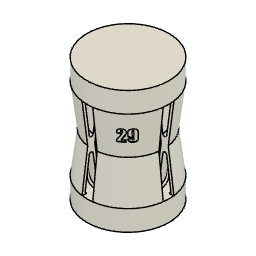
Cylinder design 3_Perez Leonardo v7 (Autodesk Fusion 360 design; units mm, degrees)
Autodesk Fusion 360 part; units mm, degrees
sketch "Sketch1" plane through (0, 0, 0) normal (0, 0, 1) x (1, 0, 0)
  line L0 (-12.7, 0) -> (12.7, 0)
  line L1 (12.7, 0) -> (12.7, 38.1)
  line L2 (12.7, 38.1) -> (-12.7, 38.1)
  line L3 (-12.7, 38.1) -> (-12.7, 0)
  line L4 (-12.7, 6.35) -> (12.7, 6.35)
  line L5 (-12.7, 31.75) -> (12.7, 31.75)
  line L6 (0, 0) -> (0, 38.1)
  line L7 (2.54, 6.35) -> (-2.54, 6.35)
  line L8 (-2.54, 6.35) -> (-2.54, 31.75)
  line L9 (-2.54, 31.75) -> (2.54, 31.75)
  line L10 (2.54, 31.75) -> (2.54, 6.35)
  line L11 (-7.62, 6.35) -> (-7.62, 31.75) construction
  line L12 (7.62, 6.35) -> (7.62, 31.75) construction
  line L13 (12.7, 19.05) -> (-12.7, 19.05) construction
  line L14 (-12.7, 6.35) -> (-11.1402, 19.0534)
  line L15 (-12.7, 6.35) -> (0.0988, 6.35) construction
  line L16 (-7.62, 6.35) -> (-9.1794, 19.05)
  line L17 (-7.62, 6.35) -> (-20.4154, 6.35) construction
  line L18 (-8.3877, 6.35) -> (-20.4994, 6.35) construction
  line L19 (-11.9323, 6.35) -> (0.0739, 6.35) construction
  line L20 (-8.3877, 6.35) -> (-9.6352, 16.51)
  line L21 (-11.9323, 6.35) -> (-10.6848, 16.51)
  line L22 (-11.9323, 31.75) -> (-10.6848, 21.59)
  line L23 (-8.3877, 31.75) -> (-9.6352, 21.59)
  line L24 (-7.62, 31.75) -> (-9.1794, 19.05)
  line L25 (-12.7, 31.75) -> (-11.1402, 19.0466)
  line L26 (-3.3077, 31.75) -> (-4.5552, 21.59)
  line L27 (-2.54, 31.75) -> (-4.0998, 19.0466)
  line L28 (-6.8523, 31.75) -> (-5.6048, 21.59)
  line L29 (-7.62, 31.75) -> (-6.0606, 19.05)
  line L30 (-2.54, 6.35) -> (-4.0998, 19.0534)
  line L31 (-7.62, 6.35) -> (-6.0606, 19.05)
  line L32 (-6.8523, 6.35) -> (-5.6048, 16.51)
  line L33 (-3.3077, 6.35) -> (-4.5552, 16.51)
  line L34 (12.7, 31.75) -> (11.1402, 19.0466)
  line L35 (11.9323, 31.75) -> (10.6848, 21.59)
  line L36 (8.3877, 31.75) -> (9.6352, 21.59)
  line L37 (7.62, 31.75) -> (9.1794, 19.05)
  line L38 (7.62, 31.75) -> (6.0606, 19.05)
  line L39 (6.8523, 31.75) -> (5.6048, 21.59)
  line L40 (3.3077, 31.75) -> (4.5552, 21.59)
  line L41 (2.54, 31.75) -> (4.0998, 19.0466)
  line L42 (2.54, 6.35) -> (4.0998, 19.0534)
  line L43 (3.3077, 6.35) -> (4.5552, 16.51)
  line L44 (6.8523, 6.35) -> (5.6048, 16.51)
  line L45 (7.62, 6.35) -> (6.0606, 19.05)
  line L46 (7.62, 6.35) -> (9.1794, 19.05)
  line L47 (8.3877, 6.35) -> (9.6352, 16.51)
  line L48 (11.9323, 6.35) -> (10.6848, 16.51)
  line L49 (12.7, 6.35) -> (11.1402, 19.0534)
  arc A0 (-9.6391, 16.51) -> (-10.6809, 16.51) centre (-10.16, 16.51) ccw
  line L50 (-10.6848, 16.51) -> (-10.6809, 16.51)
  line L51 (-9.6391, 16.51) -> (-9.6352, 16.51)
  arc A1 (-11.8606, 6.9342) -> (-11.3437, 6.35) centre (-11.3437, 6.8707) ccw
  arc A2 (-4.5591, 16.51) -> (-5.6009, 16.51) centre (-5.08, 16.51) ccw
  line L52 (-4.5552, 16.51) -> (-4.5591, 16.51)
  line L53 (-5.6009, 16.51) -> (-5.6048, 16.51)
  arc A3 (5.6009, 16.51) -> (4.5591, 16.51) centre (5.08, 16.51) ccw
  line L54 (4.5552, 16.51) -> (4.5591, 16.51)
  line L55 (5.6009, 16.51) -> (5.6048, 16.51)
  arc A4 (10.6809, 16.51) -> (9.6391, 16.51) centre (10.16, 16.51) ccw
  line L56 (10.6848, 16.51) -> (10.6809, 16.51)
  line L57 (9.6391, 16.51) -> (9.6352, 16.51)
  arc A5 (-8.9763, 6.35) -> (-8.4594, 6.9342) centre (-8.9763, 6.8707) ccw
  arc A6 (-6.7806, 6.9342) -> (-6.2637, 6.35) centre (-6.2637, 6.8707) ccw
  arc A7 (-3.8963, 6.35) -> (-3.3794, 6.9342) centre (-3.8963, 6.8707) ccw
  arc A8 (3.3794, 6.9342) -> (3.8963, 6.35) centre (3.8963, 6.8707) ccw
  arc A9 (6.2637, 6.35) -> (6.7806, 6.9342) centre (6.2637, 6.8707) ccw
  arc A10 (8.4594, 6.9342) -> (8.9763, 6.35) centre (8.9763, 6.8707) ccw
  arc A11 (11.3437, 6.35) -> (11.8606, 6.9342) centre (11.3437, 6.8707) ccw
  arc A12 (-10.6809, 21.59) -> (-9.6391, 21.59) centre (-10.16, 21.59) ccw
  line L58 (-10.6848, 21.59) -> (-10.6809, 21.59)
  line L59 (-9.6391, 21.59) -> (-9.6352, 21.59)
  line L60 (-4.5552, 21.59) -> (-4.5591, 21.59)
  line L61 (-5.6009, 21.59) -> (-5.6048, 21.59)
  arc A13 (-5.6009, 21.59) -> (-4.5591, 21.59) centre (-5.08, 21.59) ccw
  line L62 (4.5552, 21.59) -> (4.5591, 21.59)
  line L63 (5.6009, 21.59) -> (5.6048, 21.59)
  arc A14 (4.5591, 21.59) -> (5.6009, 21.59) centre (5.08, 21.59) ccw
  line L64 (10.6848, 21.59) -> (10.6809, 21.59)
  line L65 (9.6391, 21.59) -> (9.6352, 21.59)
  arc A15 (9.6391, 21.59) -> (10.6809, 21.59) centre (10.16, 21.59) ccw
  arc A16 (11.8606, 31.1658) -> (11.3437, 31.75) centre (11.3437, 31.2293) ccw
  arc A17 (8.9763, 31.75) -> (8.4594, 31.1658) centre (8.9763, 31.2293) ccw
  arc A18 (6.7806, 31.1658) -> (6.2637, 31.75) centre (6.2637, 31.2293) ccw
  arc A19 (3.8963, 31.75) -> (3.3794, 31.1658) centre (3.8963, 31.2293) ccw
  arc A20 (-3.3794, 31.1658) -> (-3.8963, 31.75) centre (-3.8963, 31.2293) ccw
  arc A21 (-6.2637, 31.75) -> (-6.7806, 31.1658) centre (-6.2637, 31.2293) ccw
  arc A22 (-8.4594, 31.1658) -> (-8.9763, 31.75) centre (-8.9763, 31.2293) ccw
  arc A23 (-11.3437, 31.75) -> (-11.8606, 31.1658) centre (-11.3437, 31.2293) ccw
  circle A24 centre (-7.62, 26.5395) radius 0.635
  circle A25 centre (-7.62, 11.5605) radius 0.635
  circle A26 centre (7.62, 11.5605) radius 0.635
  circle A27 centre (7.62, 26.5395) radius 0.635
  dimension "d1" = 25.4
  dimension "d2" = 38.1
  dimension "d3" = 6.35
  dimension "d4" = 6.35
  dimension "d5" = 25.4
  dimension "d6" = 5.08
  dimension "d7" = 5.08
  dimension "d8" = 5.08
  dimension "d9" = 83
  dimension "d10" = 83
  dimension "d11" = 83
  dimension "d12" = 83
  dimension "d13" = 0.762
  dimension "d14" = 0.762
  dimension "d15" = 10.16
  dimension "d17" = 1.0417
  dimension "d18" = 1.0414
  dimension "d49" = 1.27
  constraint horizontal L0
  constraint vertical L1
  constraint horizontal L2
  constraint vertical L3
  constraint midpoint L6.start L0
  constraint coincident L3 L4.start
  constraint coincident L1 L4.end
  constraint perpendicular L1 L4
  constraint coincident L3 L5.start
  constraint coincident L1 L5.end
  constraint perpendicular L1 L5
  constraint coincident L6.start origin
  constraint midpoint L2 L6.end
  constraint horizontal L7
  constraint vertical L8
  constraint horizontal L9
  constraint vertical L10
  constraint midpoint L4 L7
  constraint coincident L4 L11.start
  constraint coincident L5 L11.end
  constraint perpendicular L5 L11
  constraint coincident L4 L12.start
  constraint coincident L5 L12.end
  constraint perpendicular L5 L12
  constraint midpoint L1 L13.start
  constraint midpoint L3 L13.end
  constraint horizontal L15
  constraint horizontal L17
  constraint coincident L13 L16.end
  constraint horizontal L18
  constraint coincident L4 L18.start
  constraint horizontal L19
  constraint coincident L18 L19.start
  constraint perpendicular L11 L50
  constraint symmetric L4.start L13 L5.start
  constraint symmetric L11.start L13 L11.end
  constraint symmetric L13 L14.end L25.end
  constraint symmetric L13 L16.end L24.end
  constraint symmetric L13 L18.start L23.start
  constraint symmetric L13 L19.start L22.start
  constraint symmetric L13 L21.end L22.end
  constraint symmetric L13 L20.end L23.end
  constraint symmetric L4.start L11 L7.end
  constraint symmetric L16.start L11 L17.start
  constraint symmetric L11 L14.end L30.end
  constraint symmetric L11 L16.end L29.end
  constraint symmetric L11 L18.start L32.start
  constraint symmetric L11 L19.start L33.start
  constraint symmetric L11 L21.end L33.end
  constraint symmetric L11 L20.end L32.end
  constraint symmetric L11 L22.start L26.start
  constraint symmetric L11 L22.end L26.end
  constraint symmetric L11 L23.end L28.end
  constraint symmetric L11 L23.start L28.start
  constraint symmetric L11 L24.start L29.start
  constraint symmetric L11 L5.start L8.end
  constraint symmetric L11 L25.end L27.end
  constraint symmetric L4.start L6 L4.end
  constraint symmetric L6 L11.start L12.start
  constraint symmetric L6 L14.end L49.end
  constraint symmetric L6 L16.end L37.end
  constraint symmetric L6 L18.start L47.start
  constraint symmetric L6 L19.start L48.start
  constraint symmetric L6 L21.end L48.end
  constraint symmetric L6 L20.end L47.end
  constraint symmetric L6 L22.start L35.start
  constraint symmetric L6 L22.end L35.end
  constraint symmetric L6 L23.end L36.end
  constraint symmetric L6 L23.start L36.start
  constraint symmetric L6 L11.end L12.end
  constraint symmetric L6 L5.start L5.end
  constraint symmetric L6 L25.end L34.end
  constraint symmetric L6 L26.start L40.start
  constraint symmetric L6 L26.end L40.end
  constraint symmetric L6 L8.end L9.end
  constraint symmetric L6 L27.end L41.end
  constraint symmetric L6 L28.start L39.start
  constraint symmetric L6 L28.end L39.end
  constraint symmetric L6 L29.end L38.end
  constraint symmetric L6 L7.end L7.start
  constraint symmetric L6 L30.end L42.end
  constraint symmetric L6 L32.start L44.start
  constraint symmetric L6 L32.end L44.end
  constraint symmetric L6 L33.start L43.start
  constraint symmetric L6 L33.end L43.end
  constraint tangent L20 A0
  constraint tangent L21 A0
  constraint tangent L21 A1
  constraint tangent L17 A1
  constraint tangent L20 A5
  constraint tangent L18 A5
  constraint equal A1 A5
  constraint symmetric L11 A0 A2
  constraint symmetric L11 A1 A7
  constraint symmetric L11 A5 A6
  constraint symmetric L13 A0 A12
  constraint symmetric L13 A1 A23
  constraint symmetric L13 A5 A22
  constraint symmetric L13 A2 A13
  constraint symmetric L13 A7 A20
  constraint symmetric L13 A6 A21
  constraint symmetric L6 A0 A4
  constraint symmetric L6 A1 A11
  constraint symmetric L6 A5 A10
  constraint symmetric L6 A2 A3
  constraint symmetric L6 A7 A8
  constraint symmetric L6 A6 A9
  constraint symmetric L6 A18 A21
  constraint symmetric L6 A17 A22
  constraint symmetric L6 A16 A23
  constraint symmetric L6 A12 A15
  constraint symmetric L6 A13 A14
  constraint symmetric L6 A19 A20
  constraint coincident A0.start L50
  constraint collinear L50 L51
  constraint coincident A0.centre L50
  constraint coincident L4 A1.end
  constraint coincident L21 A1.start
  constraint coincident A2.end L52
  constraint collinear L52 L53
  constraint coincident A3.start L54
  constraint collinear L54 L55
  constraint coincident A4.end L56
  constraint collinear L56 L57
  constraint coincident L20 A5.end
  constraint coincident L4 A5.start
  constraint coincident L4 A6.end
  constraint coincident L32 A6.start
  constraint coincident L33 A7.end
  constraint coincident L4 A7.start
  constraint coincident L4 A8.end
  constraint coincident L43 A8.start
  constraint coincident L44 A9.end
  constraint coincident L4 A9.start
  constraint coincident L4 A10.end
  constraint coincident L47 A10.start
  constraint coincident L48 A11.end
  constraint coincident L4 A11.start
  constraint coincident A12.end L58
  constraint collinear L58 L59
  constraint collinear L60 L61
  constraint collinear L62 L63
  constraint collinear L64 L65
  constraint coincident L5 A16.end
  constraint coincident L35 A16.start
  constraint coincident L36 A17.end
  constraint coincident L5 A17.start
  constraint coincident L5 A18.end
  constraint coincident L39 A18.start
  constraint coincident L40 A19.end
  constraint coincident L5 A19.start
  constraint coincident L5 A20.end
  constraint coincident L26 A20.start
  constraint coincident L28 A21.end
  constraint coincident L5 A21.start
  constraint coincident L5 A22.end
  constraint coincident L23 A22.start
  constraint coincident L22 A23.end
  constraint coincident L5 A23.start
  constraint tangent L29 A24
  constraint tangent L24 A24
  constraint tangent L31 A25
  constraint tangent L16 A25
  constraint equal A24 A25
  constraint tangent L46 A26
  constraint tangent L45 A26
  constraint equal A25 A26
  constraint tangent L37 A27
  constraint tangent L38 A27
  constraint equal A26 A27
  measures "d1" distance of L0.start L0.end
  measures "d2" distance of L0.end L1.end
  measures "d3" distance of L2 L5
  measures "d4" distance of L0 L4
  measures "d5" distance of L7.start L9.end
  measures "d6" distance of L7.start L7.end
  measures "d7" distance of L8 L11
  measures "d8" distance of L10 L12
  measures "d9" angle of L14 L15
  measures "d10" angle of L16 L17
  measures "d11" angle of L18 L20
  measures "d12" angle of L19 L21
  measures "d13" distance of L14 L21
  measures "d14" distance of L16 L20
  measures "d15" distance of L4 L50
  measures "d17" diameter of A0
  measures "d18" diameter of A1
  measures "d49" diameter of A24
sketch "Sketch2" plane through (0, 0, 0) normal (1, 0, 0) x (0, 0, -1)
  line L0 (-7.62, 6.35) -> (-20.4154, 6.35) construction
  line L1 (-8.3877, 6.35) -> (-9.6352, 16.51)
  line L2 (-9.6391, 16.51) -> (-9.6352, 16.51)
  line L3 (-11.9323, 6.35) -> (-10.6848, 16.51)
  arc A0 (-4.5591, 16.51) -> (-5.6009, 16.51) centre (-5.08, 16.51) ccw
  arc A1 (-6.7806, 6.9342) -> (-6.2637, 6.35) centre (-6.2637, 6.8707) ccw
  arc A2 (-11.8606, 6.9342) -> (-11.3437, 6.35) centre (-11.3437, 6.8707) ccw
  arc A3 (-8.9763, 6.35) -> (-8.4594, 6.9342) centre (-8.9763, 6.8707) ccw
  line L4 (-4.5552, 16.51) -> (-4.5591, 16.51)
  arc A4 (6.2637, 6.35) -> (6.7806, 6.9342) centre (6.2637, 6.8707) ccw
  arc A5 (10.6809, 16.51) -> (9.6391, 16.51) centre (10.16, 16.51) ccw
  arc A6 (11.8606, 31.1658) -> (11.3437, 31.75) centre (11.3437, 31.2293) ccw
  line L5 (3.3077, 6.35) -> (4.5552, 16.51)
  line L6 (6.8523, 6.35) -> (5.6048, 16.51)
  line L7 (-2.54, 6.35) -> (-4.0998, 19.0534)
  line L8 (5.6009, 21.59) -> (5.6048, 21.59)
  line L9 (-7.62, 6.35) -> (-6.0606, 19.05)
  line L10 (4.5552, 16.51) -> (4.5591, 16.51)
  arc A7 (6.7806, 31.1658) -> (6.2637, 31.75) centre (6.2637, 31.2293) ccw
  arc A8 (5.6009, 16.51) -> (4.5591, 16.51) centre (5.08, 16.51) ccw
  line L11 (11.9323, 31.75) -> (10.6848, 21.59)
  line L12 (9.6391, 16.51) -> (9.6352, 16.51)
  line L13 (7.62, 31.75) -> (9.1794, 19.05)
  line L14 (2.54, 31.75) -> (2.54, 6.35)
  line L15 (5.6009, 16.51) -> (5.6048, 16.51)
  line L16 (3.3077, 31.75) -> (4.5552, 21.59)
  arc A9 (8.4594, 6.9342) -> (8.9763, 6.35) centre (8.9763, 6.8707) ccw
  line L17 (-12.7, 6.35) -> (-11.1402, 19.0534)
  line L18 (12.7, 6.35) -> (11.1402, 19.0534)
  line L19 (10.6848, 16.51) -> (10.6809, 16.51)
  line L20 (2.54, 6.35) -> (4.0998, 19.0534)
  arc A10 (4.5591, 21.59) -> (5.6009, 21.59) centre (5.08, 21.59) ccw
  arc A11 (3.8963, 31.75) -> (3.3794, 31.1658) centre (3.8963, 31.2293) ccw
  line L21 (6.8523, 31.75) -> (5.6048, 21.59)
  line L22 (7.62, 6.35) -> (9.1794, 19.05)
  line L23 (8.3877, 31.75) -> (9.6352, 21.59)
  line L24 (10.6848, 21.59) -> (10.6809, 21.59)
  line L25 (-2.54, 6.35) -> (-2.54, 31.75)
  line L26 (11.9323, 6.35) -> (10.6848, 16.51)
  line L27 (8.3877, 6.35) -> (9.6352, 16.51)
  arc A12 (9.6391, 21.59) -> (10.6809, 21.59) centre (10.16, 21.59) ccw
  arc A13 (8.9763, 31.75) -> (8.4594, 31.1658) centre (8.9763, 31.2293) ccw
  line L28 (7.62, 31.75) -> (6.0606, 19.05)
  line L29 (2.54, 31.75) -> (4.0998, 19.0466)
  line L30 (7.62, 6.35) -> (6.0606, 19.05)
  line L31 (9.6391, 21.59) -> (9.6352, 21.59)
  line L32 (4.5552, 21.59) -> (4.5591, 21.59)
  line L33 (7.62, 6.35) -> (7.62, 31.75) construction
  line L34 (12.7, 0) -> (12.7, 38.1)
  arc A14 (3.3794, 6.9342) -> (3.8963, 6.35) centre (3.8963, 6.8707) ccw
  arc A15 (11.3437, 6.35) -> (11.8606, 6.9342) centre (11.3437, 6.8707) ccw
  line L35 (0, 0) -> (0, 38.1)
  line L36 (-12.7, 38.1) -> (-12.7, 0)
  line L37 (-6.8523, 6.35) -> (-5.6048, 16.51)
  line L38 (-6.8523, 31.75) -> (-5.6048, 21.59)
  arc A16 (-8.4594, 31.1658) -> (-8.9763, 31.75) centre (-8.9763, 31.2293) ccw
  line L39 (-4.5552, 21.59) -> (-4.5591, 21.59)
  arc A17 (-5.6009, 21.59) -> (-4.5591, 21.59) centre (-5.08, 21.59) ccw
  line L40 (-3.3077, 31.75) -> (-4.5552, 21.59)
  line L41 (-9.6391, 21.59) -> (-9.6352, 21.59)
  line L42 (-8.3877, 6.35) -> (-20.4994, 6.35) construction
  line L43 (-7.62, 31.75) -> (-6.0606, 19.05)
  arc A18 (-11.3437, 31.75) -> (-11.8606, 31.1658) centre (-11.3437, 31.2293) ccw
  line L44 (-2.54, 31.75) -> (-4.0998, 19.0466)
  arc A19 (-3.8963, 6.35) -> (-3.3794, 6.9342) centre (-3.8963, 6.8707) ccw
  line L45 (-7.62, 31.75) -> (-9.1794, 19.05)
  line L46 (-12.7, 31.75) -> (-11.1402, 19.0466)
  line L47 (-11.9323, 31.75) -> (-10.6848, 21.59)
  arc A20 (-10.6809, 21.59) -> (-9.6391, 21.59) centre (-10.16, 21.59) ccw
  line L48 (-3.3077, 6.35) -> (-4.5552, 16.51)
  arc A21 (-9.6391, 16.51) -> (-10.6809, 16.51) centre (-10.16, 16.51) ccw
  line L49 (-8.3877, 31.75) -> (-9.6352, 21.59)
  arc A22 (-3.3794, 31.1658) -> (-3.8963, 31.75) centre (-3.8963, 31.2293) ccw
  line L50 (-10.6848, 21.59) -> (-10.6809, 21.59)
  line L51 (-5.6009, 16.51) -> (-5.6048, 16.51)
  line L52 (-10.6848, 16.51) -> (-10.6809, 16.51)
  line L53 (-5.6009, 21.59) -> (-5.6048, 21.59)
  arc A23 (-6.2637, 31.75) -> (-6.7806, 31.1658) centre (-6.2637, 31.2293) ccw
  line L54 (-7.62, 6.35) -> (-9.1794, 19.05)
  line L55 (-7.62, 6.35) -> (-7.62, 31.75) construction
  line L56 (-12.7, 6.35) -> (0.0988, 6.35) construction
  line L57 (2.54, 6.35) -> (-2.54, 6.35)
  line L58 (12.7, 31.75) -> (11.1402, 19.0466)
  line L59 (12.7, 38.1) -> (-12.7, 38.1)
  line L60 (-2.54, 31.75) -> (2.54, 31.75)
  line L61 (-12.7, 0) -> (12.7, 0)
  line L62 (-12.7, 31.75) -> (12.7, 31.75)
  line L63 (-11.9323, 6.35) -> (0.0739, 6.35) construction
  line L64 (12.7, 19.05) -> (-12.7, 19.05) construction
  line L65 (-12.7, 6.35) -> (12.7, 6.35)
  circle A24 centre (-7.62, 26.5395) radius 0.635
  circle A25 centre (-7.62, 11.5605) radius 0.635
  circle A26 centre (7.62, 26.5395) radius 0.635
  circle A27 centre (7.62, 11.5605) radius 0.635
  dimension "d20" = 25.4
  dimension "d21" = 38.1
  dimension "d22" = 6.35
  dimension "d23" = 6.35
  dimension "d24" = 25.4
  dimension "d25" = 5.08
  dimension "d26" = 5.08
  dimension "d27" = 5.08
  dimension "d28" = 83
  dimension "d29" = 83
  dimension "d30" = 83
  dimension "d31" = 83
  dimension "d32" = 0.762
  dimension "d33" = 0.762
  dimension "d34" = 10.16
  dimension "d35" = 1.0417
  dimension "d36" = 1.0414
  dimension "d37" = 12.7
  dimension "d50" = 1.27
  constraint horizontal L61
  constraint vertical L34
  constraint horizontal L59
  constraint vertical L36
  constraint midpoint L35.start L61
  constraint coincident L17.start L36
  constraint coincident L18.start L34
  constraint perpendicular L34 L65
  constraint coincident L46.start L36
  constraint coincident L58.start L34
  constraint perpendicular L34 L62
  constraint coincident L35.start origin
  constraint midpoint L35.end L59
  constraint horizontal L57
  constraint vertical L25
  constraint horizontal L60
  constraint vertical L14
  constraint midpoint L57 L65
  constraint coincident L0.start L65
  constraint coincident L43.start L62
  constraint perpendicular L55 L62
  constraint coincident L22.start L65
  constraint coincident L13.start L62
  constraint perpendicular L33 L62
  constraint midpoint L64.start L34
  constraint midpoint L64.end L36
  constraint horizontal L56
  constraint horizontal L0
  constraint coincident L45.end L64
  constraint horizontal L42
  constraint coincident L1.start L65
  constraint horizontal L63
  constraint coincident L3.start L42
  constraint perpendicular L52 L55
  constraint symmetric L17.start L46.start L64
  constraint symmetric L0.start L43.start L64
  constraint symmetric L17.end L46.end L64
  constraint symmetric L45.end L54.end L64
  constraint symmetric L1.start L49.start L64
  constraint symmetric L3.start L47.start L64
  constraint symmetric L3.end L47.end L64
  constraint symmetric L1.end L41.end L64
  constraint symmetric L17.start L7.start L55
  constraint symmetric L0.start L9.start L55
  constraint symmetric L17.end L7.end L55
  constraint symmetric L45.end L9.end L55
  constraint symmetric L1.start L37.start L55
  constraint symmetric L3.start L48.start L55
  constraint symmetric L3.end L4.start L55
  constraint symmetric L1.end L37.end L55
  constraint symmetric L47.start L40.start L55
  constraint symmetric L47.end L39.start L55
  constraint symmetric L41.end L38.end L55
  constraint symmetric L49.start L38.start L55
  constraint symmetric L43.start L45.start L55
  constraint symmetric L25.end L46.start L55
  constraint symmetric L46.end L44.end L55
  constraint symmetric L17.start L18.start L35
  constraint symmetric L0.start L22.start L35
  constraint symmetric L17.end L18.end L35
  constraint symmetric L45.end L13.end L35
  constraint symmetric L1.start L27.start L35
  constraint symmetric L3.start L26.start L35
  constraint symmetric L3.end L19.start L35
  constraint symmetric L1.end L12.end L35
  constraint symmetric L47.start L11.start L35
  constraint symmetric L47.end L11.end L35
  constraint symmetric L41.end L23.end L35
  constraint symmetric L49.start L23.start L35
  constraint symmetric L43.start L13.start L35
  constraint symmetric L46.start L58.start L35
  constraint symmetric L46.end L58.end L35
  constraint symmetric L40.start L16.start L35
  constraint symmetric L39.start L16.end L35
  constraint symmetric L25.end L14.start L35
  constraint symmetric L44.end L29.end L35
  constraint symmetric L38.start L21.start L35
  constraint symmetric L38.end L8.end L35
  constraint symmetric L9.end L28.end L35
  constraint symmetric L7.start L14.end L35
  constraint symmetric L7.end L20.end L35
  constraint symmetric L37.start L6.start L35
  constraint symmetric L37.end L6.end L35
  constraint symmetric L48.start L5.start L35
  constraint symmetric L4.start L5.end L35
  constraint tangent L1 A21
  constraint tangent L3 A21
  constraint tangent L3 A2
  constraint tangent L0 A2
  constraint tangent L1 A3
  constraint tangent A3 L42
  constraint equal A2 A3
  constraint symmetric A0 A21 L55
  constraint symmetric A2 A19 L55
  constraint symmetric A1 A3 L55
  constraint symmetric A20 A21 L64
  constraint symmetric A2 A18 L64
  constraint symmetric A3 A16 L64
  constraint symmetric A0 A17 L64
  constraint symmetric A19 A22 L64
  constraint symmetric A1 A23 L64
  constraint symmetric A5 L35 A21
  constraint symmetric A2 A15 L35
  constraint symmetric A3 A9 L35
  constraint symmetric A0 A8 L35
  constraint symmetric A14 L35 A19
  constraint symmetric A1 A4 L35
  constraint symmetric A7 L35 A23
  constraint symmetric A13 L35 A16
  constraint symmetric A6 L35 A18
  constraint symmetric A12 L35 A20
  constraint symmetric A10 L35 A17
  constraint symmetric A11 L35 A22
  constraint coincident L2.start L52
  constraint collinear L2 L52
  constraint coincident A21.centre L52
  constraint coincident A2.end L65
  constraint coincident A2.start L3
  constraint coincident A0.end L4
  constraint collinear L4 L51
  constraint coincident A8.start L10
  constraint collinear L10 L15
  constraint coincident A5.end L19
  constraint collinear L12 L19
  constraint coincident A3.end L1
  constraint coincident A3.start L65
  constraint coincident A1.end L65
  constraint coincident A1.start L37
  constraint coincident A19.end L48
  constraint coincident A19.start L65
  constraint coincident A14.end L65
  constraint coincident A14.start L5
  constraint coincident A4.end L6
  constraint coincident A4.start L65
  constraint coincident A9.end L65
  constraint coincident A9.start L27
  constraint coincident A15.end L26
  constraint coincident A15.start L65
  constraint coincident L41.start L50
  constraint collinear L41 L50
  constraint collinear L39 L53
  constraint collinear L8 L32
  constraint collinear L24 L31
  constraint coincident A6.end L62
  constraint coincident A6.start L11
  constraint coincident A13.end L23
  constraint coincident A13.start L62
  constraint coincident A7.end L62
  constraint coincident A7.start L21
  constraint coincident A11.end L16
  constraint coincident A11.start L62
  constraint coincident A22.end L62
  constraint coincident A22.start L40
  constraint coincident A23.end L38
  constraint coincident A23.start L62
  constraint coincident A16.end L62
  constraint coincident A16.start L49
  constraint coincident A18.end L47
  constraint coincident A18.start L62
  constraint coincident L35.start L61
  constraint tangent L43 A24
  constraint tangent L45 A24
  constraint tangent L9 A25
  constraint tangent L54 A25
  constraint equal A24 A25
  constraint tangent L28 A26
  constraint tangent L13 A26
  constraint equal A24 A26
  constraint tangent L30 A27
  constraint tangent L22 A27
  constraint equal A25 A27
  measures "d20" distance of L34.start L36.end
  measures "d21" distance of L34.start L34.end
  measures "d22" distance of L59 L62
  measures "d23" distance of L61 L65
  measures "d24" distance of L14.end L14.start
  measures "d25" distance of L14.end L7.start
  measures "d26" distance of L25 L55
  measures "d27" distance of L14 L33
  measures "d28" angle of L17 L56
  measures "d29" angle of L0 L54
  measures "d30" angle of L1 L42
  measures "d31" angle of L3 L63
  measures "d32" distance of L3 L17
  measures "d33" distance of L1 L54
  measures "d34" distance of L52 L65
  measures "d35" diameter of A21
  measures "d36" diameter of A2
  measures "d37" distance of L35.start L34
  measures "d50" diameter of A24
revolve "Revolve7" add sketch "Sketch1" angle 360 about axis through (0, 0, 0) along (0, 1, 0) second angle 360 contours L0 L1 L4 L6 L7 | L4 L5 L6 L7 L9 L10 | L4 L5 L34 L35 L36 L37 L46 L47 L48 L49 A4 L56 L57 L64 L65 A15 | L4 L5 L38 L39 L40 L41 L42 L43 L44 L45 A3 L54 L55 L62 L63 A14 | L1 L2 L5 L6 L9 | L4 L48 A11 | L4 L43 A8 | L5 L35 A16 | L5 L40 A19 | L4 L47 A10 | L4 L44 A9 | L5 L36 A17 | L5 L39 A18 | L45 L46 A26 | L37 L38 A27
revolve "Revolve8" cut sketch "Sketch1" angle 7.5 about axis through (0, 0, 0) along (0, 1, 0) second angle 7.5 contours L4 L5 L14 L16 L20 L21 L22 L23 L24 L25 A0 L50 L51 A12 L58 L59 | L4 L21 A1 | L4 L5 L34 L35 L36 L37 L46 L47 L48 L49 A4 L56 L57 L64 L65 A15 | L4 L5 L26 L27 L28 L29 L30 L31 L32 L33 A2 L52 L53 L60 L61 A13 | L4 L5 L38 L39 L40 L41 L42 L43 L44 L45 A3 L54 L55 L62 L63 A14 | L5 L22 A23 | L4 L48 A11 | L4 L33 A7 | L4 L43 A8 | L4 L20 A5 | L5 L35 A16 | L5 L26 A20 | L5 L40 A19 | L5 L23 A22 | L4 L47 A10 | L4 L32 A6 | L4 L44 A9 | L16 L31 A25 | L5 L36 A17 | L5 L28 A21 | L5 L39 A18 | L24 L29 A24 | L45 L46 A26 | L37 L38 A27
revolve "Revolve9" cut sketch "Sketch2" angle 7.5 about axis through (0, 0, 0) along (0, 1, 0) second angle 7.5 contours L1 A3 L65 | L1 L2 L3 L17 L41 L45 L46 L47 A20 A21 L49 L50 L52 L54 L62 L65 | L9 L54 A25 | A0 L4 L7 L9 L37 L38 L39 A17 L40 L43 L44 L48 L51 L53 L62 L65 | L3 A2 L65 | A1 L37 L65 | L43 L45 A24 | A19 L48 L65 | A18 L47 L62 | A16 L49 L62 | L38 A23 L62 | L5 L6 L8 L10 A8 L15 L16 L20 A10 L21 L28 L29 L30 L32 L62 L65 | A5 L11 L12 L13 L18 L19 L22 L23 L24 L26 L27 A12 L31 L58 L62 L65 | L40 A22 L62 | L5 A14 L65 | L26 A15 L65 | L16 A11 L62 | A6 L11 L62 | A4 L6 L65 | A9 L27 L65 | A7 L21 L62 | L23 A13 L62 | L22 L30 A27 | L13 L28 A26
ref_plane "WorkPlane1" through (8.3046, 25.4, 8.5514) normal (0.691487, -0.121869, 0.712035) x (0.717382, 0, -0.69668)
sketch "Sketch3" plane through (6.0408, -1.0646, 6.2203) normal (0.691487, -0.121869, 0.712035) x (0.717382, 0, -0.69668)
  line L0 (-2.327, 24.2009) -> (3.2578, 24.2009) construction
  line L1 (3.2578, 24.2009) -> (3.2578, 28.5446) construction
  line L2 (3.2578, 28.5446) -> (-2.327, 28.5446) construction
  line L3 (-2.327, 28.5446) -> (-2.327, 24.2009) construction
  dimension "d58" = 3.81
  text T0 "29" font "Impact" height 3.81 align left top in box 5.5848 x 4.3437 at (-2.327, 24.2009) x (1, 0) y (0, 1) spacing 1
extrude "Extrude1" cut sketch "Sketch3" against normal blind 0.254 text T0
